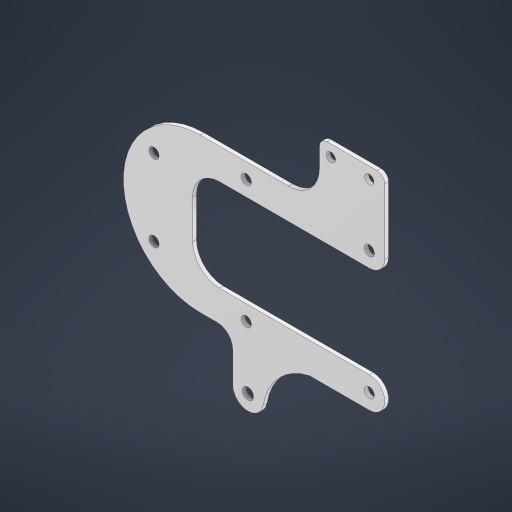
# Autodesk Inventor part: gusset
Saved by Autodesk Inventor 2024 (Build 280153000, 153)
## iProperties
Created: 2023-08-15
Part Number: gusset
Material: Acetal Resin, White
Document SubType Name: Modeling
Designer: avere
Density: 1.425 g/cm^3
Appearance: Smooth - White
Author: avere
Autodesk Inventor part; units mm, degrees
ref_plane "YZ Plane" through (0, 0, 0) normal (1, 0, 0) x (0, 1, 0)
ref_plane "XZ Plane" through (0, 0, 0) normal (0, 1, 0) x (-1, 0, 0)
ref_plane "XY Plane" through (0, 0, 0) normal (0, 0, 1) x (1, 0, 0)
sketch "Sketch1" plane through (0, 0, 0) normal (0, 0, 1) x (1, 0, 0)
  line L0 (-47.2309, 58.7326) -> (-58.3434, 58.7326)
  line L1 (-69.4559, 84.1326) -> (-69.4559, 69.8451)
  arc A0 (-69.4559, 69.8451) -> (-58.3434, 58.7326) centre (-58.3434, 69.8451) ccw
  line L2 (-69.4559, 69.8451) -> (-69.4559, 86.6091)
  line L3 (-47.2309, 96.8326) -> (-58.3434, 96.8326)
  line L4 (-69.4559, 85.7201) -> (-69.4559, 86.6091)
  arc A1 (-58.3434, 96.8326) -> (-69.4559, 85.7201) centre (-58.3434, 85.7201) ccw
  line L5 (-47.2309, 46.0326) -> (-66.2809, 46.0326)
  line L6 (-98.0309, 77.7826) -> (-98.0309, 77.7826)
  line L7 (-66.2809, 109.5326) -> (-47.2309, 109.5326)
  arc A2 (-66.2809, 109.5326) -> (-98.0309, 77.7826) centre (-66.2809, 77.7826) ccw
  arc A3 (-98.0309, 77.7826) -> (-66.2809, 46.0326) centre (-66.2809, 77.7826) ccw
  circle A4 centre (-47.2309, 103.1826) radius 2.0955
  circle A5 centre (-47.2309, 52.3826) radius 2.0955
  circle A6 centre (-85.3309, 93.5778) radius 2.0828
  circle A7 centre (-85.3309, 61.9874) radius 2.0828
  line L8 (-47.2309, 96.8326) -> (-21.8309, 96.8326)
  line L9 (-15.4809, 103.1826) -> (-15.4809, 103.1826)
  line L10 (-21.8309, 109.5326) -> (-47.2309, 109.5326)
  line L11 (-47.2309, 58.7326) -> (-21.8309, 58.7326)
  line L12 (-15.4809, 52.3826) -> (-15.4809, 52.3826)
  line L13 (-21.8309, 46.0326) -> (-47.2309, 46.0326)
  arc A8 (-15.4809, 52.3826) -> (-21.8309, 58.7326) centre (-21.8309, 52.3826) ccw
  arc A9 (-21.8309, 46.0326) -> (-15.4809, 52.3826) centre (-21.8309, 52.3826) ccw
  arc A10 (-21.8309, 96.8326) -> (-15.4809, 103.1826) centre (-21.8309, 103.1826) ccw
  arc A11 (-15.4809, 103.1826) -> (-21.8309, 109.5326) centre (-21.8309, 103.1826) ccw
  line L14 (-75.7109, 63.3494) -> (-75.7109, 92.2158)
  arc A12 (-76.923, 92.8904) -> (-76.923, 62.6748) centre (-67.5536, 77.7826) ccw
  arc A13 (-75.7109, 92.2158) -> (-76.923, 92.8904) centre (-76.5047, 92.2158) ccw
  arc A14 (-76.923, 62.6748) -> (-75.7109, 63.3494) centre (-76.5047, 63.3494) ccw
  point P0 (-69.4559, 58.7326)
  point P1 (-15.4809, 58.7326)
  point P2 (-75.7109, 93.5778)
  point P3 (-75.7109, 61.9874)
  dimension "d11" = 22.225
  dimension "d12" = 11.1125
  dimension "d13" = 11.1125
  dimension "d14" = 31.75
  dimension "d15" = 31.75
  dimension "d16" = 4.191
  dimension "d17" = 4.191
  dimension "d18" = 4.1656
  dimension "d19" = 4.1656
  dimension "d21" = 6.35
  dimension "d27" = 0.7937
  constraints: 30 end point, 24 point on circle, 20 tangent, 15 centre point, 8 point on line, 4 equal radius, 4 horizontal, 4 perpendicular, 1 collinear, 1 vertical
  measures "d11" distance of L0.start point (-69.456, 58.733)
  measures "d12" radius of A0
  measures "d13" radius of A1
  measures "d14" radius of A2
  measures "d15" radius of A3
  measures "d16" diameter of A4
  measures "d17" diameter of A5
  measures "d18" diameter of A6
  measures "d19" diameter of A7
  measures "d21" radius of A8
  measures "d27" radius of A13
extrude "Extrusion1" add sketch "Sketch1" along normal blind 1.5875 contours L11 A8 A9 L13 L5 A3 A2 L7 L10 A11 A10 L8 L3 A1 L2 L1 A0 L0 | A14 A12 A13 L14
sketch "Sketch2" plane through (-21.8309, 46.0326, 1.5875) normal (0, 0, 1) x (1, 0, 0)
  circle A0 centre (-24.7079, -19.05) radius 2.3114
  arc A1 (-31.0579, -19.05) -> (-18.4424, -20.0828) centre (-24.7079, -19.05) ccw
  line L0 (-31.0579, -19.05) -> (-31.0579, -6.35)
  line L1 (-44.45, 0) -> (0, 0) projected
  arc A2 (-31.0579, -6.35) -> (-37.4079, 0) centre (-37.4079, -6.35) ccw
  arc A3 (0, 0) -> (0, 12.7) centre (0, 6.35) ccw projected
  arc A4 (1.2054, 0.1155) -> (-18.4424, -20.0828) centre (5.886, -24.0929) ccw
  circle A5 centre (25.4, 6.35) radius 2.0955
  line L2 (0, 63.5) -> (-44.45, 63.5) projected
  arc A6 (0, 50.8) -> (0, 63.5) centre (0, 57.15) ccw projected
  arc A7 (25.4, 0) -> (25.4, 12.7) centre (25.4, 6.35) ccw
  line L3 (0, 12.7) -> (25.4, 12.7)
  line L4 (0, 0) -> (25.4, 0)
  circle A8 centre (25.4, 57.15) radius 2.0955
  arc A9 (25.4, 50.8) -> (25.4, 63.5) centre (25.4, 57.15) ccw
  line L5 (25.4, 50.8) -> (0, 50.8)
  line L6 (0, 63.5) -> (25.4, 63.5)
  arc A10 (0, 50.8) -> (0, 63.5) centre (0, 57.15) ccw projected
  point P0 (21.8309, -46.0326)
  point P1 (-31.0579, 0)
  point P2 (0.6434, 0)
  dimension "d22" = 4.6228
  dimension "d24" = 6.35
  dimension "d29" = 4.191
  dimension "d31" = 4.191
  dimension "d32" = 12.7
  constraints: 12 point on circle, 10 end point, 9 tangent, 8 centre point, 3 coincident, 2 horizontal, 1 point on line, 1 vertical, 1 other
  measures "d22" diameter of A0
  measures "d24" radius of A2
  measures "d29" diameter of A5
  measures "d31" diameter of A8
  measures "d32" diameter of A9
extrude "Extrusion2" add sketch "Sketch2" against normal blind 1.5875
sketch "Sketch5" plane through (3.5691, 103.1826, 0) normal (0, 0, -1) x (-1, 0, 0)
  line L0 (0, 6.35) -> (69.85, 6.35) projected
  line L1 (12.7, 0) -> (20.6375, 0) construction
  arc A0 (69.85, -57.15) -> (69.85, 6.35) centre (69.85, -25.4) ccw projected
  line L2 (69.85, 6.35) -> (50.8, 6.35)
  line L3 (0, 6.35) -> (0, 6.35)
  circle A1 centre (15.875, 25.4) radius 1.905
  arc A2 (0, 6.35) -> (0, -6.35) centre (0, 0) ccw projected
  line L4 (-6.35, 0) -> (-6.35, 26.9875)
  circle A3 centre (0, 25.4) radius 1.905
  line L5 (-3.175, 30.1625) -> (15.875, 30.1625)
  line L6 (20.6375, 19.05) -> (20.6375, 26.9875)
  line L7 (17.4625, 30.1625) -> (15.875, 30.1625)
  arc A4 (20.6375, 26.9875) -> (17.4625, 30.1625) centre (17.4625, 26.9875) ccw
  arc A5 (-3.175, 30.1625) -> (-6.35, 26.9875) centre (-3.175, 26.9875) ccw
  line L8 (33.3375, 6.35) -> (50.8, 6.35)
  arc A6 (20.6375, 19.05) -> (33.3375, 6.35) centre (33.3375, 19.05) ccw
  point P0 (3.5691, -103.1826)
  point P1 (12.7, 30.1625)
  point P2 (12.7, 6.35)
  point P3 (20.6375, 6.35)
  point P4 (33.3375, 6.35)
  dimension "d33" = 30.1625
  dimension "d37" = 3.81
  dimension "d41" = 3.81
  dimension "d42" = 3.175
  dimension "d43" = 12.7
  constraints: 16 end point, 7 point on circle, 7 tangent, 6 point on line, 5 centre point, 2 collinear, 2 vertical, 1 equal radius, 1 horizontal, 1 perpendicular
  measures "d33" distance of L1.start point (12.7, 30.162)
  measures "d37" diameter of A1
  measures "d41" diameter of A3
  measures "d42" radius of A4
  measures "d43" radius of A6
extrude "Extrusion3" add sketch "Sketch5" against normal blind 1.5875
body "Solid1"
